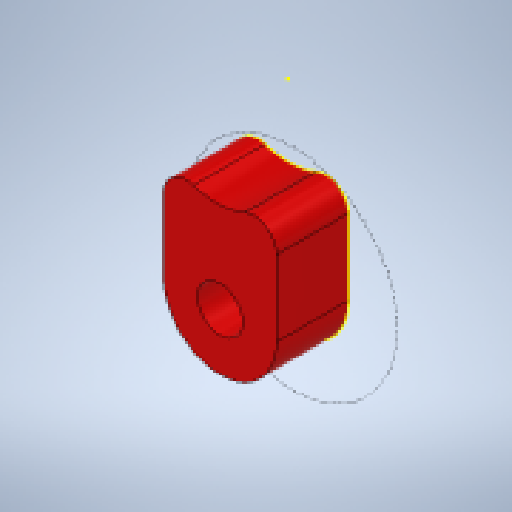
# Autodesk Inventor part: Cam - Lever
Saved by Autodesk Inventor 2023.2 (Build 272271000, 271)
## iProperties
Created: 2024-01-19
Part Number: Cam - Lever
Material: Nylon 6/6
Document SubType Name: Modeling
Designer: Nathan Cai
Density: 1.13 g/cm^3
Appearance: Red
Mass: 0.32887 g
Surface Area: 3.14473 cm^2
Volume: 0.291035 cm^3
Author: Nathan Cai
Autodesk Inventor part; units mm, degrees
ref_plane "YZ Plane" through (0, 0, 0) normal (1, 0, 0) x (0, 1, 0)
ref_plane "XZ Plane" through (0, 0, 0) normal (0, 1, 0) x (-1, 0, 0)
ref_plane "XY Plane" through (0, 0, 0) normal (0, 0, 1) x (1, 0, 0)
sketch "Sketch1" plane through (0, 0, 0) normal (0, 0, 1) x (1, 0, 0)
  circle A0 centre (0, 0) radius 1.5
  circle A1 centre (0, 0) radius 3.75
  circle A2 centre (0, 0) radius 6 construction
  line L0 (0, 0) -> (0, 6) construction
  circle A3 centre (-0.25, 10.7596) radius 4.7625
  line L1 (0, 0) -> (0, 6) construction
  line L2 (3.75, 0) -> (3.75, 6)
  line L3 (-3.75, 6) -> (-3.75, 0)
  arc A4 (-3.75, 0) -> (3.75, 0) centre (0, 0) ccw
  arc A5 (3.75, 6) -> (-2.25, 3) centre (0, 6) ccw
  arc A6 (-3.6447, 0.8824) -> (-3.6447, 5.1176) centre (-12.392, 3) ccw
  point P0 (0, 3)
  point P1 (-3.6798, 6.7221)
  point P2 (3.75, 0)
  point P3 (3.3637, 7.6576)
  point P4 (-3.75, 0)
  point P5 (-3.5189, 7.2961)
  dimension "d2" = 12
  dimension "d0" = 3
  dimension "d1" = 7.5
  dimension "d3" = 9.525
  dimension "d4" = 3.75
  dimension "d9" = 0.25
  dimension "d10" = 9
  constraints: 11 point on circle, 10 end point, 6 centre point, 6 tangent, 3 coincident, 2 equal length, 1 midpoint, 1 vertical, 1 vertical alignment, 3 other
  measures "d0" diameter of A0
  measures "d1" diameter of A1
  measures "d3" diameter of A3
  measures "d4" radius of A5
  measures "d9" distance from line of L0 A3.centre
  measures "d10" radius of A6
extrude "Extrusion1" add sketch "Sketch1" along normal blind 4.7625 contours A1 | A1 A5 A3 L2 | A1 A6 A5 | L3 A5 A6 A1
fillet "Fillet1" radius 1.5 2 edges at (3.3637, 7.6576, 2.3813) (-3.5189, 7.2961, 2.3813)
sketch "Sketch2" plane through (0, 0, 0) normal (0, 0, -1) x (-1, 0, 0)
  line L0 (-3.75, 0) -> (-3.75, 5.0177) projected
  arc A0 (-3.75, 0) -> (3.75, 0) centre (0, 0) ccw projected
  circle A1 centre (0, 0) radius 1.5 projected
  circle A2 centre (0, 0) radius 6.9991 construction
  arc A3 (3.75, 4.825) -> (1.771, 6.2465) centre (2.25, 4.825) ccw projected
  arc A4 (-1.6512, 6.393) -> (1.771, 6.2465) centre (0.25, 10.7596) ccw projected
  arc A5 (-1.6512, 6.393) -> (-3.75, 5.0177) centre (-2.25, 5.0177) ccw projected
  line L1 (3.75, 4.825) -> (3.75, 0) projected
  arc A6 (-1.6512, 6.393) -> (-3.75, 5.0177) centre (-2.25, 5.0177) ccw projected
  constraints: 1 centre point, 1 coincident, 1 tangent
equation "\"d4\" = 0.5 * d1"
body "Solid1"
